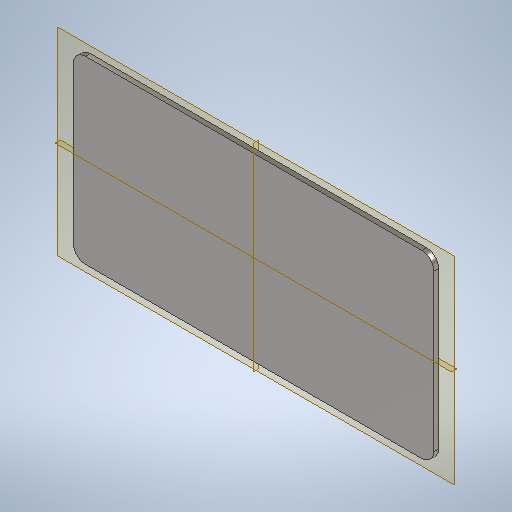
# Autodesk Inventor part: Sessao_28_03_001_001
Saved by Autodesk Inventor 2026 (Build 300175000, 175)
## iProperties
Created: 2025-03-28
Part Number: Sessao_28_03_001_001
Material: Steel, Galvanized
Document SubType Name: Sheet Metal
Designer: Carlos Dias
Density: 7.85 g/cm^3
Sheet Metal Rule: Default
Appearance: Galvanized
Author: Carlos Dias
Autodesk Inventor part; units mm, degrees
sketch "Sketch1" plane through (0, 0, 0) normal (0, 0, 1) x (1, 0, 0)
  line L0 (-750, 375) -> (750, 375)
  line L1 (750, 375) -> (750, -375)
  line L2 (750, -375) -> (-750, -375)
  line L3 (-750, -375) -> (-750, 375)
  line L4 (-750, 375) -> (750, -375) construction
  line L5 (750, 375) -> (-750, -375) construction
  point P0 (0, 0)
  dimension "d0" = 1500
  dimension "d1" = 750
  constraints: 12 end point, 2 midpoint, 2 parallel, 1 horizontal, 1 perpendicular
  measures "d0" distance of L0.start L0.end
  measures "d1" distance of L2.end L0.start
extrude "Extrusion1" add sketch "Sketch1" along normal mid plane 20
fillet "Fillet1" radius 50 4 edges at (-750, 375, 0) (750, 375, 0) (750, -375, 0) (-750, -375, 0)
equation "\"BendRadius\" = Thickness"
equation "\"BendReliefWidth\" = Thickness"
equation "\"BendReliefDepth\" = 0.5 * Thickness"
equation "\"CornerReliefSize\" = 4 * Thickness"
equation "\"MinimumRemnant\" = 2 * Thickness"
equation "\"TransitionRadius\" = BendRadius"
equation "\"JacobiRadiusSize\" = BendRadius"
equation "\"GapSize\" = Thickness"
equation "\"Thickness\" = 3.048"
body "Solid1"
